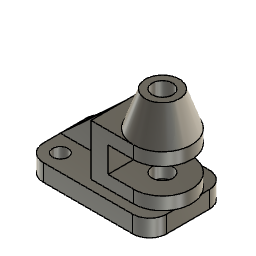
MACHANICAL TASK_PAVIN v1 (Autodesk Fusion 360 design; units mm, degrees)
Autodesk Fusion 360 part; units mm, degrees
sketch "Sketch1" plane through (0, 0, 0) normal (0, 0, 1) x (1, 0, 0)
  line L0 (20, 0) -> (125, 0)
  line L1 (145, 20) -> (145, 70)
  line L2 (125, 90) -> (20, 90)
  line L3 (0, 70) -> (0, 20)
  arc A0 (20, 90) -> (0, 70) centre (20, 70) ccw
  arc A1 (0, 20) -> (20, 0) centre (20, 20) ccw
  arc A2 (125, 0) -> (145, 20) centre (125, 20) ccw
  arc A3 (145, 70) -> (125, 90) centre (125, 70) ccw
  circle A4 centre (20, 70) radius 9
  circle A5 centre (20, 20) radius 9
  point P0 (145, 90)
  point P1 (0, 90)
  dimension "d1" = 145
  dimension "d3" = 20
  dimension "d4" = 50
  dimension "d5" = 18
  dimension "d6" = 18
  constraint horizontal L0
  constraint vertical L1
  constraint horizontal L2
  constraint vertical L3
  constraint coincident P1 L2
  constraint coincident P1 L3
  constraint tangent L2 A0
  constraint tangent L3 A0
  constraint coincident origin L0
  constraint coincident origin L3
  constraint tangent L0 A1
  constraint tangent L3 A1
  constraint equal A0 A1
  constraint tangent L0 A2
  constraint tangent L1 A2
  constraint equal A0 A2
  constraint coincident P0 L1
  constraint coincident P0 L2
  constraint tangent L1 A3
  constraint tangent L2 A3
  constraint equal A0 A3
  constraint concentric A0 A4
  constraint concentric A1 A5
  measures "d1" distance of P0 P1
  measures "d3" radius of A0
  measures "d4" distance of L3.start L3.end
  measures "d5" diameter of A4
  measures "d6" diameter of A5
extrude "Extrude1" add sketch "Sketch1" along normal blind 20
sketch "Sketch2" plane through (0, 0, 20) normal (0, 0, 1) x (-1, 0, 0)
  circle A0 centre (-20, -70) radius 9
  circle A1 centre (-20, -20) radius 9
  arc A2 (-145, -70) -> (-125, -90) centre (-125, -70) ccw
  line L0 (-125, -90) -> (-20, -90)
  arc A3 (-20, -90) -> (0, -70) centre (-20, -70) ccw
  line L1 (0, -70) -> (0, -20)
  arc A4 (0, -20) -> (-20, 0) centre (-20, -20) ccw
  line L2 (-20, 0) -> (-125, 0)
  arc A5 (-125, 0) -> (-145, -20) centre (-125, -20) ccw
  line L3 (-145, -20) -> (-145, -70)
  line L4 (-65, -50) -> (-65, -79)
  line L5 (-65, -79) -> (-115, -79)
  line L6 (-115, -79) -> (-115, -79)
  line L7 (-65, -11) -> (-65, -40)
  line L8 (0, -40) -> (-65, -40)
  line L9 (-65, -50) -> (0, -50)
  line L10 (0, -50) -> (0, -40)
  line L11 (0, -40) -> (-65, -50) construction
  line L12 (-65, -40) -> (0, -50) construction
  line L13 (-65, -11) -> (-115, -11)
  line L14 (-115, -11) -> (-115, -79)
  point P0 (-135, -79)
  dimension "d11" = 50
  dimension "d22" = 29
  constraint perpendicular L4 L5
  constraint coincident P0 L6
  constraint horizontal L8
  constraint parallel L8 L9
  constraint coincident L1 L8.start
  constraint perpendicular L7 L13
  constraint perpendicular L5 L14
  measures "d11" distance of L4.end L5.end
  measures "d22" distance of L7.start L7.end
extrude "Extrude2" add sketch "Sketch2" along normal blind 60 contours L1 L4 L5 L7 L8 L9 L10 L13 L14
sketch "Sketch3" plane through (0, 0, 0) normal (0, 1, 0) x (1, 0, 0)
  line L0 (0, -20) -> (65, -80)
  line L1 (65, -80) -> (0, -80)
  line L2 (0, -80) -> (0, -20)
  line L3 (135, -35) -> (85, -35)
  line L4 (85, -35) -> (85, -65)
  line L5 (85, -65) -> (135, -65)
  line L6 (135, -65) -> (135, -35)
  point P0 (65, -20)
  dimension "d18" = 20
  dimension "d19" = 15
  constraint horizontal L1
  constraint perpendicular L1 L2
  constraint perpendicular L2 L3
  constraint perpendicular L1 L4
  constraint perpendicular L2 L5
  constraint perpendicular L3 L6
  measures "d18" distance of L0.end L4
  measures "d19" distance of L0.end L5
form "Form1" [no effect]
extrude "Extrude3" cut sketch "Sketch3" along normal through all
ref_plane "WorkPlane1" through (0, 45, 0) normal (0, 1, 0) x (0, 0, 1)
sketch "Sketch7" plane through (0, 45, 0) normal (0, 1, 0) x (1, 0, 0)
  line L0 (115, -80) -> (115, -120)
  line L1 (115, -120) -> (95, -120)
  line L2 (95, -120) -> (81, -80)
  line L3 (81, -80) -> (115, -80)
  dimension "d24" = 40
  dimension "d25" = 20
  dimension "d26" = 34
  constraint vertical L0
  constraint perpendicular L0 L1
  constraint perpendicular L0 L3
  measures "d24" distance of L0.start L0.end
  measures "d25" distance of L0.end L1.end
  measures "d26" distance of L0.start L2.end
revolve "Revolve1" add sketch "Sketch7" angle 360 about axis through (115, 45, 80) along (0, 0, 1)
sketch "Sketch8" plane through (0, 0, 80) normal (0, 0, -1) x (1, 0, 0)
  line L0 (115, -11) -> (115, -79)
  arc A0 (115, -79) -> (115, -11) centre (115, -45) ccw
  line L1 (115, -79) -> (115, -11)
  arc A1 (115, -79) -> (115, -11) centre (115, -45) ccw
  constraint concentric A0 A1
  constraint coincident L0.end A0.start
  constraint coincident L0.start A0.end
extrude "Extrude4" add sketch "Sketch8" along normal up to surface (60 mm away)
sketch "Sketch9" plane through (0, 0, 0) normal (0, 1, 0) x (1, 0, 0)
  line L0 (115, -65) -> (150, -65)
  line L1 (150, -65) -> (150, -35)
  line L2 (150, -35) -> (115, -35)
  line L3 (115, -35) -> (115, -65)
  dimension "d30" = 35
  dimension "d31" = 30
  constraint horizontal L0
  constraint vertical L1
  constraint horizontal L2
  constraint vertical L3
  measures "d30" distance of L0.start L0.end
  measures "d31" distance of L0.start L2.end
extrude "Extrude5" cut sketch "Sketch9" along normal through all
sketch "Sketch10" plane through (0, 0, 120) normal (0, 0, 1) x (-1, 0, 0)
  circle A0 centre (-115, -45) radius 20
  circle A1 centre (-115, -45) radius 12
  dimension "d33" = 24
  constraint concentric A0 A1
  measures "d33" diameter of A1
extrude "Extrude6" cut sketch "Sketch10" against normal up to surface (100 mm away) contours A1
equation "d22 = 34 mm - 5 mm"
equation "d23 = ( 90 / 2 ) * 1 mm"
equation "d26 = ( 68 / 2 ) * 1 mm"
